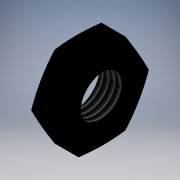
# Autodesk Inventor part: C96S32_NUT
Saved by Autodesk Inventor 2017.3 (Build 213256000, 256)
## iProperties
Part Number: C96S32_NUT
Material: Generic
Catalog Web Link: www.cadenas.de
Description: C96 NUT-ISO Cylinder:Standard Double Acting,Single/Double Rod
Vendor: SMC
Document SubType Name: Modeling
Designer: partserver
Manufacturer: SMC
Mass: 1.12156 g
Surface Area: 8.52563 cm^2
Volume: 1.12156 cm^3
Density: 1 g/cm^3
Appearance: PSOLRGB-0-0-0
Category: PARTsolutions
Company: SMC
Title: C96S32_NUT
Author: Cadenas PARTsolutions
Comments: ISO Cylinder:Standard Double Acting,Single/Double Rod
PSOL_IDENT_0: {$CADENAS_DATA\23d-libs\smc_jp\actuator\standard_air_cylinder\cp96_c96\c96\parts\c96_nut.prj},174 {V
PSOL_IDENT_1: TYP=3D},{NB=C96S32_NUT},{LINA=C96S32_NUT},{NN=C96 NUT},{DATE=05.07.2021 01:48:07},{GEOMDATE=23.04.20
PSOL_IDENT_2: 12 00:00:00},{VERSION=v090415094912},{LINEID=20},{WBVAR=},{WBNUMERIC=}  {NB=C96S32_NUT},{LINA=C96S32
PSOL_IDENT_3: _NUT},{KT=DUMMY},{BORE=32},{KK=M10x1.25},{KRA=10},{KRP=1.25},{H=6},{B=17}
NB: C96S32_NUT
NN: C96 NUT
NT: ISO Cylinder:Standard Double Acting,Single/Double Rod
NBSYN: C96S$BORE._NUT
LINA: C96S32_NUT
CATALOG: SMC (JP
BORE: 32
KK: M10x1.25
H: 6
B: 17
SUPPLIER: SMC
ARTICLENO: C96S32_NUT
BOMINFO: C96S32_NUT
CREATOR: CADENAS GmbH
Autodesk Inventor part; units mm, degrees
sketch "Sketch_2" plane through (0, 0, 0) normal (0, 0, 1) x (1, 0, 0)
  line L0 (3, 0) -> (-3, 0)
  line L1 (-3, 8) -> (-3, 5)
  line L2 (-3, 5) -> (-2.3235, 4.3235)
  line L3 (-2.3235, 4.3235) -> (2.3235, 4.3235)
  line L4 (2.3235, 4.3235) -> (3, 5)
  line L5 (3, 5) -> (3, 8)
  line L6 (3, 8) -> (1.955, 11.9)
  line L7 (1.955, 11.9) -> (-1.955, 11.9)
  line L8 (-1.955, 11.9) -> (-3, 8)
  constraints: 18 end point
revolve "Revolution1" add sketch "Sketch_2" angle 360 about axis through (3, 0, 0) along (1, 0, 0)
thread "Thread1" size "M10x1.25" class "6H" standard "ISO Metric profile" full length
sketch "Sketch_3" plane through (0, 0, 0) normal (1, 0, 0) x (0, 1, 0)
  circle A0 centre (0, 0) radius 17
  line L0 (-4.9075, 8.5) -> (-9.815, 0)
  line L1 (-9.815, 0) -> (-4.9075, -8.5)
  line L2 (-4.9075, -8.5) -> (4.9075, -8.5)
  line L3 (4.9075, -8.5) -> (9.815, 0)
  line L4 (9.815, 0) -> (4.9075, 8.5)
  line L5 (4.9075, 8.5) -> (-4.9075, 8.5)
  constraints: 12 end point, 1 centre point
extrude "Extrusion1" cut sketch "Sketch_3" along normal mid plane 6
ref_plane "NUT_ROD_XY" through (0, 0, 0) normal (1, 0, 0) x (0, 0, -1)
ref_plane "NUT_ROD_YZ" through (0, 0, 0) normal (0, 0, -1) x (0, 1, 0)
ref_plane "NUT_ROD_ZX" through (0, 0, 0) normal (0, 1, 0) x (1, 0, 0)
body "Solid1"
